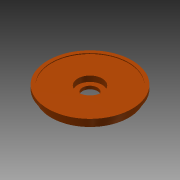
# Autodesk Inventor part: Upper Thermal Barrier
Saved by Autodesk Inventor 2015 (Build 190159000, 159)
## iProperties
Created: 2015-12-03
Part Number: Upper Thermal Barrier
Material: Phenolic Resin
Document SubType Name: Modeling
Designer: Jared
Density: 1.38 g/cm^3
Appearance: Smooth - Light Orange
Author: Jared
Autodesk Inventor part; units mm, degrees
ref_plane "YZ Plane" through (0, 0, 0) normal (1, 0, 0) x (0, 1, 0)
ref_plane "XZ Plane" through (0, 0, 0) normal (0, 1, 0) x (-1, 0, 0)
ref_plane "XY Plane" through (0, 0, 0) normal (0, 0, 1) x (1, 0, 0)
sketch "Sketch1" plane through (0, 0, 0) normal (0, 0, 1) x (1, 0, 0)
  line L0 (-12.7, 0) -> (-65.8749, 0)
  line L1 (-65.8749, 0) -> (-65.8749, 6.985)
  line L2 (-71.4375, 9.525) -> (-65.8749, 9.525)
  line L3 (-65.8749, 9.525) -> (-63.6397, 9.525)
  line L4 (-63.6397, 9.525) -> (-63.6397, 6.985)
  line L5 (-63.6397, 6.985) -> (-65.8749, 6.985)
  line L6 (-65.5002, 14.605) -> (-20.701, 14.605)
  line L7 (-12.7, 5.2578) -> (-20.701, 5.2578)
  line L8 (-20.701, 5.2578) -> (-20.701, 14.605)
  line L9 (-12.7, 5.2578) -> (-12.7, 0)
  line L10 (0, 14.605) -> (0, 0)
  line L11 (-71.4375, 15.875) -> (-65.5002, 15.875)
  line L12 (-65.5002, 15.875) -> (-65.5002, 14.605)
  line L13 (-71.4375, 15.875) -> (-71.4375, 9.525)
  dimension "d0" = 65.8749
  dimension "d1" = 9.525
  dimension "d7" = 2.54
  dimension "d8" = 2.2352
  dimension "d9" = 6.985
  dimension "d24" = 9.3472
  dimension "d25" = 5.2578
  dimension "d26" = 8.001
  dimension "d27" = 12.7
  dimension "d28" = 5.2578
  dimension "d30" = 5.9372
  dimension "d32" = 6.35
  dimension "d33" = 1.27
  dimension "d34" = 44.7992
  constraints: 28 end point, 5 perpendicular, 3 horizontal, 3 vertical, 1 parallel, 1 point on line
  measures "d0" distance of L10.end L0.end
  measures "d1" distance of L0.end L2.end
  measures "d7" distance of L3.end L4.end
  measures "d8" distance of L4.end L1.end
  measures "d9" distance of L0.end L1.end
  measures "d24" distance of L7.end L6.end
  measures "d25" distance of L7.start L0.start
  measures "d26" distance of L7.start L7.end
  measures "d27" distance from line of L10.end L9
  measures "d28" distance from line of L10.end L7
  measures "d30" distance of L11.start L11.end
  measures "d32" distance of L11.start L2.start
  measures "d33" distance of L11.end L6.start
  measures "d34" distance of L6.start L6.end
revolve "Revolution2" add sketch "Sketch1" angle 360 about axis through (0, 14.605, 0) along (0, -1, 0)
body "Solid2"
